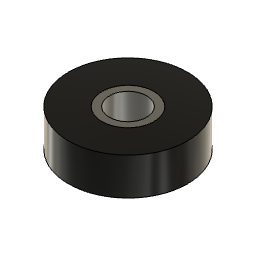
ers_bot (Autodesk Fusion 360 archive; units mm, degrees)
design "bearing"
Autodesk Fusion 360 part; units mm, degrees
sketch "Sketch1" plane through (0, 0, 0) normal (0, 0, 1) x (1, 0, 0) in component "inner bearing"
  circle A0 centre (0, 0) radius 3.5
  circle A1 centre (0, 0) radius 2.5
  dimension "d1" = 5
  dimension "d2" = 1
  constraint coincident A0.centre A1.centre
  constraint concentric A0 A1
  measures "d1" diameter of A1
  measures "d2" distance of A0 A1
extrude "Extrude1" add sketch "Sketch1" along normal blind 5 makes body 1 in component "inner bearing"
sketch "Sketch1 (2)" plane through (0, 0, 0) normal (0, 0, 1) x (1, 0, 0) in component "outer bearing"
  circle A0 centre (0, 0) radius 8
  circle A1 centre (0, 0) radius 3.5
  dimension "d5" = 16
  constraint coincident A0.centre A1.centre
  measures "d5" diameter of A0
extrude "Extrude1'" add sketch "Sketch1 (2)" along normal up to surface (5 mm away) separate body makes body 2 in component "outer bearing"
component "inner bearing" placed x (1, 0, 0) y (0, 1, 0) z (0, 0, 1) at (0, 0, 0)
component "outer bearing" placed x (1, 0, 0) y (0, 1, 0) z (0, 0, 1) at (0, 0, 0)
